Autodesk Fusion 360 part; units mm, degrees
(part 2 of 2)
sketch "Sketch2 (3)" plane through (0, 500, 0) normal (0, -1, 0) x (1, 0, 0) in component "Inner Rotor Generator"
  line L0 (100, 994.9874) -> (100, 3598.6108)
  arc A0 (100, 3598.6108) -> (-100, 3598.6108) centre (0, 0) ccw
  line L1 (-100, 3598.6108) -> (-100, 994.9874)
  arc A1 (-100, 994.9874) -> (-410.8912, 911.6844) centre (0, 0) ccw
  line L2 (-410.8912, 911.6844) -> (-1712.7029, 3166.4884)
  arc A2 (-1712.7029, 3166.4884) -> (-1885.908, 3066.4884) centre (0, 0) ccw
  line L3 (-1885.908, 3066.4884) -> (-584.0963, 811.6844)
  arc A3 (-584.0963, 811.6844) -> (-811.6844, 584.0963) centre (0, 0) ccw
  line L4 (-811.6844, 584.0963) -> (-3066.4884, 1885.908)
  arc A4 (-3066.4884, 1885.908) -> (-3166.4884, 1712.7029) centre (0, 0) ccw
  line L5 (-3166.4884, 1712.7029) -> (-911.6844, 410.8912)
  arc A5 (-911.6844, 410.8912) -> (-994.9874, 100) centre (0, 0) ccw
  line L6 (-994.9874, 100) -> (-3598.6108, 100)
  arc A6 (-3598.6108, 100) -> (-3598.6108, -100) centre (0, 0) ccw
  line L7 (-3598.6108, -100) -> (-994.9874, -100)
  arc A7 (-994.9874, -100) -> (-911.6844, -410.8912) centre (0, 0) ccw
  line L8 (-911.6844, -410.8912) -> (-3166.4884, -1712.7029)
  arc A8 (-3166.4884, -1712.7029) -> (-3066.4884, -1885.908) centre (0, 0) ccw
  line L9 (-3066.4884, -1885.908) -> (-811.6844, -584.0963)
  arc A9 (-811.6844, -584.0963) -> (-584.0963, -811.6844) centre (0, 0) ccw
  line L10 (-584.0963, -811.6844) -> (-1885.908, -3066.4884)
  arc A10 (-1885.908, -3066.4884) -> (-1712.7029, -3166.4884) centre (0, 0) ccw
  line L11 (-1712.7029, -3166.4884) -> (-410.8912, -911.6844)
  arc A11 (-410.8912, -911.6844) -> (-100, -994.9874) centre (0, 0) ccw
  line L12 (-100, -994.9874) -> (-100, -3598.6108)
  arc A12 (-100, -3598.6108) -> (100, -3598.6108) centre (0, 0) ccw
  line L13 (100, -3598.6108) -> (100, -994.9874)
  arc A13 (100, -994.9874) -> (410.8912, -911.6844) centre (0, 0) ccw
  line L14 (410.8912, -911.6844) -> (1712.7029, -3166.4884)
  arc A14 (1712.7029, -3166.4884) -> (1885.908, -3066.4884) centre (0, 0) ccw
  line L15 (1885.908, -3066.4884) -> (584.0963, -811.6844)
  arc A15 (584.0963, -811.6844) -> (811.6844, -584.0963) centre (0, 0) ccw
  line L16 (811.6844, -584.0963) -> (3066.4884, -1885.908)
  arc A16 (3066.4884, -1885.908) -> (3166.4884, -1712.7029) centre (0, 0) ccw
  line L17 (3166.4884, -1712.7029) -> (911.6844, -410.8912)
  arc A17 (911.6844, -410.8912) -> (994.9874, -100) centre (0, 0) ccw
  line L18 (994.9874, -100) -> (3598.6108, -100)
  arc A18 (3598.6108, -100) -> (3598.6108, 100) centre (0, 0) ccw
  line L19 (3598.6108, 100) -> (994.9874, 100)
  arc A19 (994.9874, 100) -> (911.6844, 410.8912) centre (0, 0) ccw
  line L20 (911.6844, 410.8912) -> (3166.4884, 1712.7029)
  arc A20 (3166.4884, 1712.7029) -> (3066.4884, 1885.908) centre (0, 0) ccw
  line L21 (3066.4884, 1885.908) -> (811.6844, 584.0963)
  arc A21 (811.6844, 584.0963) -> (584.0963, 811.6844) centre (0, 0) ccw
  line L22 (584.0963, 811.6844) -> (1885.908, 3066.4884)
  arc A22 (1885.908, 3066.4884) -> (1712.7029, 3166.4884) centre (0, 0) ccw
  line L23 (1712.7029, 3166.4884) -> (410.8912, 911.6844)
  arc A23 (410.8912, 911.6844) -> (100, 994.9874) centre (0, 0) ccw
delete_face "DeleteFace1" 1 faces at (499.3785, 1833.3333, -24.9229) on bodies 2 in component "Inner Rotor Generator"
sketch "Sketch5" plane through (0, 500, 0) normal (0, -1, 0) x (1, 0, 0)
  circle A0 centre (0, 0) radius 1000
  constraint coincident A0.centre origin
extrude "Extrude5'" add sketch "Sketch5" along normal blind 11000 and the other way blind 4000 bodies 2 in component "Inner Rotor Generator"
sketch "Sketch6" plane through (0, 0, 0) normal (1, 0, 0) x (0, 1, 0)
component "Inner Rotor Generator" placed x (1, 0, 0) y (0, 1, 0) z (0, 0, 1) at (-9696.4454, 4500, -183.4467)
component "Hub" placed x (1, 0, 0) y (0, 1, 0) z (0, 0, 1) at (-9696.4454, 0, -183.4467)
